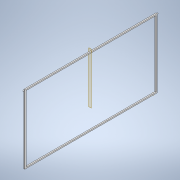
# Autodesk Inventor part: porta1
Saved by Autodesk Inventor 2022 (Build 260153000, 153)
## iProperties
Created: 2022-08-29
Part Number: porta1
Material: Generic
Document SubType Name: Modeling
Designer: cvss2
Density: 1 g/cm^3
Appearance: Default
portaLargura: 470,000 mm
portaAltura: 1138,000 mm
Author: cvss2
Autodesk Inventor part; units mm, degrees
ref_plane "YZ Plane" through (0, 0, 0) normal (1, 0, 0) x (0, 1, 0)
ref_plane "XZ Plane" through (0, 0, 0) normal (0, 1, 0) x (-1, 0, 0)
ref_plane "XY Plane" through (0, 0, 0) normal (0, 0, 1) x (1, 0, 0)
sketch "Sketch1" plane through (0, 0, 0) normal (1, 0, 0) x (0, 1, 0)
  line L0 (0, 0) -> (-490, 0)
  line L1 (-490, 0) -> (-490, -1138)
  line L2 (-490, -1138) -> (0, -1138)
  line L3 (0, -1138) -> (0, 0)
  line L4 (-480, -1128) -> (-480, -10)
  line L5 (-480, -10) -> (-10, -10)
  line L6 (-10, -10) -> (-10, -1128)
  line L7 (-10, -1128) -> (-480, -1128)
  dimension "d0" = 490
  dimension "portaAltura" = 1138
  dimension "d2" = 10
  dimension "portaLargura" = 470
  constraints: 16 end point, 4 parallel, 2 perpendicular, 1 horizontal, 3 other
  measures "d0" distance of L2.end L1.end
  measures "portaAltura" distance of L1.end L0.end
  measures "d2" distance between parallel lines of L1 L4
  measures "portaLargura" distance of L6.end L4.start
extrude "Extrusion1" add sketch "Sketch1" along normal blind 10
sketch "Sketch2" plane through (0, -490, 0) normal (0, 0, 1) x (1, 0, 0)
  line L0 (0, 490) -> (0, 0) projected
  line L1 (0, 0) -> (10, 0) projected
  line L2 (10, 490) -> (10, 0) projected
  line L3 (0, 490) -> (10, 490) projected
  line L4 (0, 0) -> (-3.182, -3.182)
  line L5 (0, 0) -> (4.5, 0) construction
  line L6 (0, 490) -> (0, 0) projected
  circle A0 centre (-3.182, -3.182) radius 5
  circle A1 centre (-3.182, -3.182) radius 4
  dimension "d5" = 4.5
  dimension "d6" = 135
  dimension "d7" = 1
  dimension "d10" = 10
  constraints: 4 end point, 2 centre point, 1 coincident, 1 equal length, 1 horizontal
  measures "d5" distance of L0.end L4.end
  measures "d6" angle of L4 L5
  measures "d7" radial gap between concentric circles of A0 A1
  measures "d10" diameter of A0
extrude "Extrusion2" [suppressed]
ref_plane "Work Plane1" through (0, 0, -569) normal (0, 0, 1) x (1, 0, 0)
mirror "Mirror1" [suppressed]
fillet "Fillet1" [suppressed]
ref_plane "Work Plane2" through (0, -490, -1113) normal (0, 0, 1) x (1, 0, 0)
sketch "Sketch3" plane through (0, -490, -1113) normal (0, 0, 1) x (1, 0, 0)
  arc A0 (0, 0.6748) -> (0.6748, 0) centre (-3.182, -3.182) ccw projected
  circle A1 centre (-3.182, -3.182) radius 4 projected
  line L0 (0.6748, 0) -> (10, 0) projected
  circle A2 centre (-3.182, -3.182) radius 5
  point P0 (0, 490)
  point P1 (0, 0.6748)
  constraints: 1 coincident, 3 other
extrude "Extrusion3" [suppressed]
sketch "Sketch4" plane through (0, 0, 0) normal (0, 0, 1) x (1, 0, 0)
  circle A0 centre (-3.182, -493.182) radius 4 projected
  arc A1 (0, -489.3252) -> (0.6748, -490) centre (-3.182, -493.182) ccw projected
  circle A2 centre (-3.182, -493.182) radius 4 projected
  line L0 (0, -490) -> (10, -490) projected
  circle A3 centre (-3.182, -493.182) radius 5
  point P0 (0, 0)
  point P1 (0, -489.3252)
  constraints: 1 coincident, 3 other
extrude "Extrusion4" [suppressed]
sketch "Sketch5" plane through (0, -490, -35) normal (0, 0, -1) x (-1, 0, 0)
  circle A0 centre (3.182, -3.182) radius 4 projected
  arc A1 (-0.6748, 0) -> (0, 0.6748) centre (3.182, -3.182) ccw projected
  circle A2 centre (3.182, -3.182) radius 5
  point P0 (0, 490)
  point P1 (0, 0.6748)
  constraints: 1 coincident, 3 other
extrude "Extrusion5" [suppressed]
sketch "Sketch6" plane through (0, 0, 0) normal (0, 0, 1) x (1, 0, 0)
  line L0 (0, -490) -> (10, -490) projected
  line L1 (10, 0) -> (10, -490) projected
  line L2 (0, 0) -> (10, 0) projected
  line L3 (0, 0) -> (0, -490) projected
  line L4 (10, -490) -> (10, 0) construction
  line L5 (0, -10) -> (10, -10) construction
  line L6 (10, 0) -> (0, -10) construction
  line L7 (0, 0) -> (10, 0) construction
  line L8 (0, 0) -> (10, -10) construction
  circle A0 centre (5, -5) radius 2.5
  dimension "d19" = 5
  constraints: 4 end point, 1 centre point, 1 midpoint
  measures "d19" diameter of A0
extrude "Extrusion6" [suppressed]
sketch "Sketch7" plane through (5, -5, 10) normal (0, 0, 1) x (1, 0, 0)
  circle A0 centre (0, 0) radius 2.5 projected
  circle A1 centre (0, 0) radius 5
  point P0 (-5, 5)
  dimension "d22" = 10
  constraints: 1 centre point, 1 coincident
  measures "d22" diameter of A1
extrude "Extrusion7" [suppressed]
mirror "Mirror2" [suppressed]
body "Solid1"
